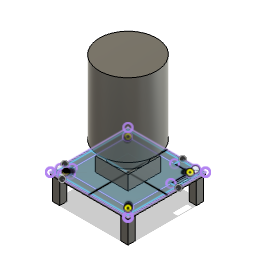
camera_base (Autodesk Fusion 360 archive; units mm, degrees)
design "rgb_cam"
Autodesk Fusion 360 part; units mm, degrees
sketch "スケッチ1" plane through (0, 0, 0) normal (0, 1, 0) x (1, 0, 0)
sketch "スケッチ2" plane through (0, 0, 0) normal (0, 1, 0) x (1, 0, 0)
  line L0 (-19, 19) -> (19, 19)
  line L1 (19, 19) -> (19, -19)
  line L2 (19, -19) -> (-19, -19)
  line L3 (-19, -19) -> (-19, 19)
  line L4 (-19, 19) -> (19, -19) construction
  line L5 (19, 19) -> (-19, -19) construction
  line L6 (-8, 8) -> (8, -8) construction
  line L7 (8, 8) -> (-8, -8) construction
  dimension "d5" = 38
  dimension "d6" = 38
  dimension "d7" = 16
  dimension "d8" = 16
  constraint horizontal L0
  constraint perpendicular L0 L1
  constraint parallel L0 L2
  constraint parallel L1 L3
  constraint coincident L4 origin
  constraint coincident L5 origin
  constraint coincident L6 origin
  constraint coincident L7 origin
  measures "d5" distance of L1.end L2.end
  measures "d6" distance of L0.end L1.end
  measures "d7" distance of L6.end L7.end
  measures "d8" distance of L7.start L6.end
extrude "押し出し1" add sketch "スケッチ2" along normal blind 1.2
sketch "スケッチ3" plane through (0, 1.2, 0) normal (0, 1, 0) x (-1, 0, 0)
  line L0 (19, 19) -> (-19, 19)
  line L1 (-19, 19) -> (-19, -19)
  line L2 (-19, -19) -> (19, -19)
  line L3 (19, -19) -> (19, 19)
  line L4 (8, -8) -> (-8, -8)
  line L5 (-8, -8) -> (-8, 8)
  line L6 (-8, 8) -> (8, 8)
  line L7 (8, 8) -> (8, -8)
  line L8 (8, -8) -> (-8, 8) construction
  line L9 (-8, -8) -> (8, 8) construction
  dimension "d11" = 16
  dimension "d12" = 16
  constraint horizontal L4
  constraint perpendicular L4 L5
  constraint parallel L4 L6
  constraint parallel L5 L7
  constraint coincident L8 origin
  constraint coincident L9 origin
  measures "d11" distance of L5.end L6.end
  measures "d12" distance of L4.end L5.end
extrude "押し出し2" add sketch "スケッチ3" along normal blind 7 contours L4 L5 L6 L7
sketch "スケッチ4" plane through (0, 8.2, 0) normal (0, 1, 0) x (-1, 0, 0)
  line L0 (8, 8) -> (-8, 8)
  line L1 (-8, 8) -> (-8, -8)
  line L2 (-8, -8) -> (8, -8)
  line L3 (8, -8) -> (8, 8)
  circle A0 centre (0, 0) radius 8
  dimension "d15" = 16
  constraint coincident A0.centre origin
  measures "d15" diameter of A0
extrude "押し出し3" add sketch "スケッチ4" along normal blind 7 contours A0
sketch "スケッチ5" plane through (0, 15.2, 0) normal (0, 1, 0) x (-1, 0, 0)
  circle A0 centre (0, 0) radius 8
  circle A1 centre (0, 0) radius 14
  dimension "d18" = 28
  constraint coincident A0.centre A1.centre
  measures "d18" diameter of A1
extrude "押し出し4" add sketch "スケッチ5" along normal blind 36 contours A0 | A1
sketch "スケッチ6" plane through (0, 0, 0) normal (1, 0, 0) x (0, 0, -1)
sketch "スケッチ7" plane through (0, 1.2, 0) normal (0, 1, 0) x (-1, 0, 0)
  line L0 (8, 8) -> (8, -8)
  line L1 (8, -8) -> (-8, -8)
  line L2 (-8, -8) -> (-8, 8)
  line L3 (-8, 8) -> (8, 8)
  line L4 (19, 19) -> (-19, 19)
  line L5 (-19, 19) -> (-19, -19)
  line L6 (-19, -19) -> (19, -19)
  line L7 (19, -19) -> (19, 19)
sketch "スケッチ8" plane through (0, 1.2, 0) normal (0, 1, 0) x (-1, 0, 0)
sketch "スケッチ9" plane through (0, 1.2, 0) normal (0, 1, 0) x (-1, 0, 0)
  line L0 (-18, 18) -> (18, 18)
  line L1 (18, 18) -> (18, -18)
  line L2 (18, -18) -> (-18, -18)
  line L3 (-18, -18) -> (-18, 18)
  constraint horizontal L0
  constraint vertical L1
  constraint horizontal L2
  constraint vertical L3
sketch "スケッチ10" plane through (0, 1.2, 0) normal (0, 1, 0) x (-1, 0, 0)
  line L0 (-18, 18) -> (18, 18)
  line L1 (-18, -18) -> (-18, 18)
  circle A0 centre (-16.75, 16.75) radius 1.25
  circle A1 centre (-16.75, 16.75) radius 1.25
  line L2 (18, -18) -> (-18, -18)
  circle A2 centre (-16.75, -16.75) radius 1.25
  line L3 (18, 18) -> (18, -18)
  circle A3 centre (16.75, 16.75) radius 1.25
  circle A4 centre (16.75, -16.75) radius 1.25
  dimension "d24" = 1.25
  dimension "d25" = 1.25
  dimension "d26" = 1.25
  dimension "d27" = 1.25
  dimension "d28" = 1.25
  constraint tangent L0 A0
  constraint tangent L1 A0
  constraint tangent L1 A2
  constraint tangent L2 A2
  constraint tangent L0 A3
  constraint tangent L3 A3
  constraint tangent L2 A4
  constraint tangent L3 A4
  measures "d24" radius of A0
  measures "d25" radius of A1
  measures "d26" radius of A2
  measures "d27" radius of A3
  measures "d28" radius of A4
hole "穴1" at (-16.75, 1.2, 16.75) at (-16.75, 1.2, -16.75) at (16.75, 1.2, 16.75) at (16.75, 1.2, -16.75) direction (0, -1, 0) diameter 2.5 end through all
sketch "スケッチ11" plane through (0, 0, 0) normal (0, -1, 0) x (1, 0, 0)
  circle A0 centre (16.75, 16.75) radius 1.25
  circle A1 centre (-16.75, 16.75) radius 1.25
  circle A2 centre (-16.75, -16.75) radius 1.25
  circle A3 centre (16.75, -16.75) radius 1.25
  line L0 (19, 19) -> (-19, 19)
  line L1 (-19, 19) -> (-19, -19)
  line L2 (-19, -19) -> (19, -19)
  line L3 (19, -19) -> (19, 19)
  line L4 (18.5, -15) -> (15, -15)
  line L5 (15, -15) -> (15, -18.5)
  line L6 (15, -18.5) -> (18.5, -18.5)
  line L7 (18.5, -18.5) -> (18.5, -15)
  line L8 (-15, -15) -> (-18.5, -15)
  line L9 (-18.5, -15) -> (-18.5, -18.5)
  line L10 (-18.5, -18.5) -> (-15, -18.5)
  line L11 (-15, -18.5) -> (-15, -15)
  line L12 (-15, 18.5) -> (-18.5, 18.5)
  line L13 (-18.5, 18.5) -> (-18.5, 15)
  line L14 (-18.5, 15) -> (-15, 15)
  line L15 (-15, 15) -> (-15, 18.5)
  line L16 (18.5, 18.5) -> (15, 18.5)
  line L17 (15, 18.5) -> (15, 15)
  line L18 (15, 15) -> (18.5, 15)
  line L19 (18.5, 15) -> (18.5, 18.5)
  dimension "d32" = 3.5
  dimension "d33" = 3.5
  dimension "d34" = 3.5
  dimension "d35" = 3.5
  dimension "d36" = 3.5
  dimension "d37" = 3.5
  dimension "d38" = 3.5
  constraint horizontal L4
  constraint vertical L5
  constraint horizontal L6
  constraint vertical L7
  constraint horizontal L8
  constraint vertical L9
  constraint horizontal L10
  constraint vertical L11
  constraint horizontal L12
  constraint vertical L13
  constraint horizontal L14
  constraint vertical L15
  constraint horizontal L16
  constraint vertical L17
  constraint horizontal L18
  constraint vertical L19
  measures "d32" distance of L4.start L6.end
  measures "d33" distance of L8.start L8.end
  measures "d34" distance of L8.start L10.end
  measures "d35" distance of L12.start L12.end
  measures "d36" distance of L12.start L14.end
  measures "d37" distance of L16.start L16.end
  measures "d38" distance of L16.start L18.end
extrude "押し出し5" add sketch "スケッチ11" along normal blind 11.2 contours L4 L5 L6 L7 | L8 L9 L10 L11 | L12 L13 L14 L15 | L16 L17 L18 L19
sketch "スケッチ12" plane through (0, 1.2, 0) normal (0, 1, 0) x (-1, 0, 0)
  line L0 (-19, -19) -> (19, -19)
  line L1 (0, -19) -> (0, -15.2)
  line L2 (-19, 19) -> (-19, -19)
  line L3 (-19, 0) -> (-15.2, 0)
  line L4 (-15.2, 0) -> (0, 0)
  line L5 (0, 0) -> (0, -15.2)
  line L6 (19, 19) -> (-19, 19)
  line L7 (0, 19) -> (0, 15.2)
  line L8 (19, -19) -> (19, 19)
  line L9 (19, 0) -> (15.2, 0)
  line L10 (15.2, 0) -> (0, 0)
  line L11 (0, 0) -> (0, 15.2)
  dimension "d41" = 3.8
  dimension "d42" = 3.8
  dimension "d43" = 3.8
  dimension "d44" = 3.8
  constraint midpoint L0 L1.start
  constraint perpendicular L0 L1
  constraint midpoint L2 L3.start
  constraint perpendicular L2 L3
  constraint horizontal L4
  constraint vertical L5
  constraint midpoint L6 L7.start
  constraint perpendicular L6 L7
  constraint midpoint L8 L9.start
  constraint horizontal L10
  constraint vertical L11
  measures "d41" distance of L1.start L1.end
  measures "d42" distance of L3.start L3.end
  measures "d43" distance of L7.start L7.end
  measures "d44" distance of L9.start L9.end
sketch "スケッチ13" plane through (0, 1.2, 0) normal (0, 1, 0) x (-1, 0, 0)
  point P0 (15.2, -15.2)
  point P1 (15.2, 15.2)
  point P2 (-15.2, 15.2)
  point P3 (-15.2, -15.2)
sketch "スケッチ14" plane through (0, 1.2, 0) normal (0, 1, 0) x (-1, 0, 0)
  point P0 (-15.2, -15.2)
  point P1 (-15.2, 15.2)
sketch "スケッチ15" plane through (0, 1.2, 0) normal (0, 1, 0) x (-1, 0, 0)
sketch "スケッチ16" plane through (0, 1.2, 0) normal (0, 1, 0) x (-1, 0, 0)
  line L0 (-18, -13) -> (-16, -13)
  line L1 (-16, -13) -> (-16, -4)
  line L2 (-16, -4) -> (-18, -4)
  line L3 (-18, -4) -> (-18, -13)
  line L4 (-18, -18) -> (-18, 18)
  line L5 (-18, -13) -> (-16, -13)
  line L6 (-16, -13) -> (-16, -4)
  line L7 (-16, -4) -> (-18, -4)
  line L8 (-18, -4) -> (-18, -13)
  dimension "d65" = 2
  dimension "d66" = 9
  constraint horizontal L0
  constraint vertical L1
  constraint horizontal L2
  constraint vertical L3
  constraint coincident L0.start L4
  constraint horizontal L5
  constraint vertical L6
  constraint horizontal L7
  constraint vertical L8
  measures "d65" distance of L0.start L0.end
  measures "d66" distance of L0.start L2.end
sketch "スケッチ17" plane through (0, 1.2, 0) normal (0, 1, 0) x (-1, 0, 0)
  line L0 (-18, -13) -> (-16, -13)
  line L1 (-16, -13) -> (-16, -6.3929)
  line L2 (-16, -6.3929) -> (-18, -6.3929)
  line L3 (-18, -6.3929) -> (-18, -13)
  line L4 (-18, -18) -> (-18, 18)
  dimension "d67" = 2
  constraint horizontal L0
  constraint vertical L1
  constraint horizontal L2
  constraint vertical L3
  constraint coincident L0.start L4
  measures "d67" distance of L0.start L0.end
extrude "押し出し7" cut sketch "スケッチ17" against normal blind 2
sketch "スケッチ18" plane through (0, 1.2, 0) normal (0, 1, 0) x (-1, 0, 0)
  line L0 (-19, -19) -> (19, -19)
  line L1 (-7.8161, -19) -> (-7.8161, -15)
  line L2 (-7.8161, -15) -> (-15.8248, -15)
  line L3 (-19, 19) -> (-19, -19)
  line L4 (-19, -5.7602) -> (-15.3, -5.7602)
  line L5 (-15.3, -5.7602) -> (-15.3, -17.7602)
  dimension "d70" = 4
  dimension "d72" = 3.7
  dimension "d73" = 12
  constraint coincident L0 L1.start
  constraint perpendicular L0 L1
  constraint perpendicular L1 L2
  constraint coincident L3 L4.start
  constraint perpendicular L3 L4
  constraint perpendicular L4 L5
  measures "d70" distance of L1.start L1.end
  measures "d72" distance of L4.start L4.end
  measures "d73" distance of L4.end L5.end
sketch "スケッチ19" plane through (0, 1.2, 0) normal (0, 1, 0) x (-1, 0, 0)
  line L0 (19, 19) -> (-19, 19)
  line L1 (13.2678, 19) -> (13.2678, 15)
  line L2 (19, -19) -> (19, 19)
  line L3 (19, 12.0237) -> (15.3, 12.0237)
  line L4 (15.3, 12.0237) -> (15.3, 17.0237)
  line L5 (13.2678, 15) -> (18.2678, 15)
  dimension "d74" = 4
  dimension "d75" = 3.7
  dimension "d76" = 5
  dimension "d77" = 5
  constraint coincident L0 L1.start
  constraint coincident L2 L3.start
  constraint perpendicular L2 L3
  constraint perpendicular L3 L4
  constraint perpendicular L2 L5
  measures "d74" distance of L1.start L1.end
  measures "d75" distance of L3.start L3.end
  measures "d76" distance of L3.end L4.end
  measures "d77" distance of L1.end L5.end
sketch "スケッチ20" plane through (0, 1.2, 0) normal (0, 1, 0) x (-1, 0, 0)
  line L0 (15.3, 15) -> (-15.3, 15)
  line L1 (-15.3, 15) -> (-15.3, -15)
  line L2 (-15.3, -15) -> (15.3, -15)
  line L3 (15.3, -15) -> (15.3, 15)
  line L4 (15.3, 12.0237) -> (15.3, 17.0237)
  line L5 (13.2678, 15) -> (18.2678, 15)
  line L6 (-7.8161, -15) -> (-15.8248, -15)
  line L7 (-15.3, -5.7602) -> (-15.3, -17.7602)
  constraint horizontal L0
  constraint vertical L1
  constraint horizontal L2
  constraint vertical L3
  constraint coincident L1.end L6
  constraint coincident L1.end L7
  constraint coincident L0.start L4
  constraint coincident L0.start L5
sketch "スケッチ21" plane through (0, 1.2, 0) normal (0, 1, 0) x (-1, 0, 0)
  line L0 (-15.3, -5.7602) -> (-15.3, -17.7602)
  line L1 (-15.3, -15) -> (15.3, -15)
  circle A0 centre (-14.16, -13.86) radius 1.14
  line L2 (-15.3, 15) -> (-15.3, -15)
  line L3 (15.3, 15) -> (-15.3, 15)
  circle A1 centre (-14.16, 13.86) radius 1.14
  line L4 (15.3, -15) -> (15.3, 15)
  circle A2 centre (14.16, 13.86) radius 1.14
  circle A3 centre (14.16, -13.86) radius 1.14
  dimension "d78" = 1.14
  dimension "d79" = 1.14
  dimension "d80" = 1.14
  dimension "d81" = 1.14
  constraint tangent L0 A0
  constraint tangent L1 A0
  constraint tangent L2 A1
  constraint tangent L3 A1
  constraint tangent L3 A2
  constraint tangent L4 A2
  constraint tangent L1 A3
  constraint tangent L4 A3
  measures "d78" radius of A0
  measures "d79" radius of A1
  measures "d80" radius of A2
  measures "d81" radius of A3

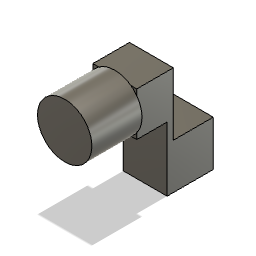
design "thermal_cam"
Autodesk Fusion 360 part; units mm, degrees
sketch "スケッチ1" plane through (0, 0, 0) normal (0, 1, 0) x (1, 0, 0)
sketch "スケッチ2" plane through (0, 0, 0) normal (0, 1, 0) x (1, 0, 0)
  line L0 (-15.5737, 13.3531) -> (5.4263, 13.3531)
  line L1 (5.4263, 13.3531) -> (5.4263, -8.7469)
  line L2 (5.4263, -8.7469) -> (-15.5737, -8.7469)
  line L3 (-15.5737, -8.7469) -> (-15.5737, 13.3531)
  dimension "d1" = 21
  dimension "d2" = 22.1
  constraint horizontal L0
  constraint vertical L1
  constraint horizontal L2
  constraint vertical L3
  measures "d1" distance of L0.start L0.end
  measures "d2" distance of L0.start L2.end
extrude "押し出し1" add sketch "スケッチ2" along normal blind 21.7
sketch "スケッチ3" plane through (0, 21.7, 0) normal (0, 1, 0) x (-1, 0, 0)
  line L0 (15.5737, 8.7469) -> (-5.4263, 8.7469)
  line L1 (-5.4263, 8.7469) -> (-5.4263, -13.3531)
  line L2 (-5.4263, -13.3531) -> (15.5737, -13.3531)
  line L3 (15.5737, -13.3531) -> (15.5737, 8.7469)
  line L4 (15.5737, 8.7469) -> (-5.4263, 8.7469)
  line L5 (-5.4263, 8.7469) -> (-5.4263, 5.7469)
  line L6 (-5.4263, 5.7469) -> (15.5737, 5.7469)
  line L7 (15.5737, 5.7469) -> (15.5737, 8.7469)
  dimension "d5" = 21
  dimension "d6" = 3
  constraint horizontal L4
  constraint vertical L5
  constraint horizontal L6
  constraint vertical L7
  constraint coincident L0.start L3.end
  measures "d5" distance of L0.start L0.end
  measures "d6" distance of L0.start L6.end
sketch "スケッチ4" plane through (0, 21.7, 0) normal (0, 1, 0) x (-1, 0, 0)
extrude "押し出し2" add sketch "スケッチ3" along normal blind 30.01 contours L0 L1 L3 L4 L5 L6 L7
sketch "スケッチ5" plane through (0, 0, 8.7469) normal (0, 0, 1) x (1, 0, 0)
  line L0 (-15.5737, 0) -> (5.4263, 0)
  line L1 (5.4263, 0) -> (5.4263, 51.71)
  line L2 (5.4263, 51.71) -> (-15.5737, 51.71)
  line L3 (-15.5737, 51.71) -> (-15.5737, 0)
  line L4 (-15.5737, 51.71) -> (5.4263, 51.71)
  line L5 (5.4263, 51.71) -> (5.4263, 30.71)
  line L6 (5.4263, 30.71) -> (-15.5737, 30.71)
  line L7 (-15.5737, 30.71) -> (-15.5737, 51.71)
  dimension "d9" = 21
  constraint horizontal L4
  constraint vertical L5
  constraint horizontal L6
  constraint vertical L7
  constraint coincident L2.end L3.start
  measures "d9" distance of L2.end L6.end
extrude "押し出し3" add sketch "スケッチ5" along normal blind 14.5 contours L1 L2 L3 L4 L5 L6 L7
sketch "スケッチ6" plane through (0, 0, 23.2469) normal (0, 0, 1) x (1, 0, 0)
  line L0 (-15.5737, 30.71) -> (5.4263, 30.71)
  line L1 (5.4263, 30.71) -> (5.4263, 51.71)
  line L2 (5.4263, 51.71) -> (-15.5737, 51.71)
  line L3 (-15.5737, 51.71) -> (-15.5737, 30.71)
  circle A0 centre (-5.0737, 41.21) radius 13
  dimension "d12" = 26
  measures "d12" diameter of A0
extrude "押し出し4" add sketch "スケッチ6" along normal blind 24 contours L0 L1 L2 L3 A0 | L0 A0 | L3 A0 | L1 A0 | L2 A0
